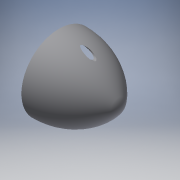
# Autodesk Inventor part: Cabeza
Saved by Autodesk Inventor 2018.3 (Build 223284000, 284)
## iProperties
Created: 2019-03-20
Part Number: Cabeza
Material: Generic
Document SubType Name: Modeling
Designer: Mario
Density: 1 g/cm^3
Appearance: Default
Mass: 6.88146 g
Surface Area: 140.288 cm^2
Volume: 6.88146 cm^3
Author: Mario
Autodesk Inventor part; units mm, degrees
ref_plane "YZ Plane" through (0, 0, 0) normal (1, 0, 0) x (0, 1, 0)
ref_plane "XZ Plane" through (0, 0, 0) normal (0, 1, 0) x (-1, 0, 0)
ref_plane "XY Plane" through (0, 0, 0) normal (0, 0, 1) x (1, 0, 0)
sketch "Sketch1" plane through (0, 0, 0) normal (0, 0, 1) x (1, 0, 0)
  line L0 (0, 0) -> (0, 29)
  line L1 (0, 0) -> (48.0517, 0)
  arc A0 (50, 0) -> (46.0452, 6.0087) centre (0, -28.6034) ccw construction
  arc A1 (0, 29) -> (50, 0) centre (0, -28.6034) ccw construction
  line L2 (0, -29) -> (0, 29) construction
  arc A2 (48.0517, 0) -> (46.0452, 6.0087) centre (38.0517, 0) ccw
  arc A3 (28.0517, 0) -> (48.0517, 0) centre (38.0517, 0) ccw construction
  arc A4 (46.0452, 6.0087) -> (28.0517, 0) centre (38.0517, 0) ccw construction
  arc A5 (46.0452, 6.0087) -> (0, 29) centre (0, -28.6034) ccw
  line L3 (48.0517, 0) -> (50, 0) construction
  dimension "d2" = 57.6035
  dimension "d16" = 50
  dimension "d18" = 58
  dimension "d21" = 11.9483
  dimension "d22" = 10
  dimension "d23" = 28.0517
  constraints: 12 point on circle, 6 centre point, 6 end point, 2 coincident, 2 horizontal, 1 point on line, 1 vertical, 1 vertical alignment
  measures "d2" radius of A0
  measures "d16" distance of L0.start L3.end
  measures "d18" distance of L2.start L2.end
  measures "d21" distance of point (38.052, 0) L3.end
  measures "d22" radius of A2
  measures "d23" distance from line of A3.start L2
revolve "Revolution1" add sketch "Sketch1" angle 360 about axis through (0, 0, 0) along (1, 0, 0)
ref_plane "Work Plane1" through (50, 0, 0) normal (-1, 0, 0) x (0, 0, 1)
shell "Shell1" thickness 1 removed faces 1 at (0, 5.4913, -3.3287)
sketch "Sketch2" plane through (50, 0, 0) normal (-1, 0, 0) x (0, 0, 1)
  circle A0 centre (0, 0) radius 29 projected
  line L0 (29, 0) -> (-29, 0) construction
  point P0 (-24, 0)
  point P1 (24, 0)
  dimension "d19" = 5
  dimension "d20" = 5
  constraints: 2 end point, 2 horizontal alignment, 2 point on circle, 1 horizontal, 1 point on line
  measures "d19" distance of point (24, 0) L0.start
  measures "d20" distance of L0.end point (-24, 0)
hole "Hole1" at (50, 0, -24) at (50, 0, 24) direction (-1, 0, 0) diameter 5 end through all
equation "\"d16\" = L"
equation "\"d21\" = X_o"
equation "\"d20\" = d19"
equation "\"R\" = 0.5 * d18"
equation "\"L\" = 50"
equation "\"Rho\" = 1"
equation "\"X_o\" = 11.948311"
body "Solid1"
